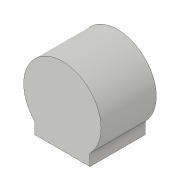
# Autodesk Inventor part: Part6
Saved by Autodesk Inventor 2017 (Build 210142000, 142)
## iProperties
Created: 2017-05-11
Part Number: Part6
Material: Generic
Document SubType Name: Modeling
Designer: zallen
Density: 1 g/cm^3
Appearance: Default
Author: zallen
Autodesk Inventor part; units mm, degrees
ref_plane "YZ Plane" through (0, 0, 0) normal (1, 0, 0) x (0, 1, 0)
ref_plane "XZ Plane" through (0, 0, 0) normal (0, 1, 0) x (-1, 0, 0)
ref_plane "XY Plane" through (0, 0, 0) normal (0, 0, 1) x (1, 0, 0)
sketch "Sketch1" plane through (0, 0, 0) normal (0, 0, 1) x (1, 0, 0)
  circle A0 centre (0, 0) radius 35
  dimension "d0" = 70
  constraints: 1 centre point, 1 coincident
  measures "d0" diameter of A0
extrude "Extrusion1" add sketch "Sketch1" along normal mid plane 50
sketch "Sketch2" plane through (0, 0, 0) normal (0, 0, 1) x (1, 0, 0)
  circle A0 centre (0, 0) radius 35 projected
  line L0 (0, -35) -> (25, -35)
  line L1 (25, -35) -> (25, -24.4949)
  arc A1 (0, -35) -> (25, -24.4949) centre (0, 0) ccw
  line L2 (25, -24.4949) -> (-25, -24.4949)
  line L3 (-25, -35) -> (0, -35)
  line L4 (-25, -35) -> (-25, -24.4949)
  arc A2 (-25, -24.4949) -> (0, -35) centre (0, 0) ccw
  dimension "d3" = 25
  dimension "d6" = 25
  constraints: 10 end point, 9 point on circle, 3 tangent, 2 centre point, 2 concentric, 2 horizontal, 1 parallel, 1 perpendicular, 1 vertical
  measures "d3" distance of L0.start L0.end
  measures "d6" distance from line of L3.end L4
extrude "Extrusion2" add sketch "Sketch2" along normal mid plane 50
body "Solid1"
